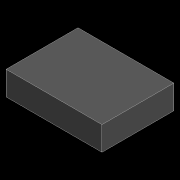
# Autodesk Inventor part: RecieverMockup
Saved by Autodesk Inventor 2022 (Build 260153000, 153)
## iProperties
Created: 2022-09-26
Part Number: RecieverMockup
Material: Generic
Document SubType Name: Modeling
Designer: tandu
Density: 1 g/cm^3
Appearance: Generic
RecieverLongSide: 0.50000000 in
RecieverShortSide: 0.37500000 in
RecieverThickness: 0.12500000 in
Author: tandu
Autodesk Inventor part; units mm, degrees
ref_plane "YZ Plane" through (0, 0, 0) normal (1, 0, 0) x (0, 1, 0)
ref_plane "XZ Plane" through (0, 0, 0) normal (0, 1, 0) x (-1, 0, 0)
ref_plane "XY Plane" through (0, 0, 0) normal (0, 0, 1) x (1, 0, 0)
sketch "Sketch1" plane through (0, 0, 0) normal (0, 1, 0) x (-1, 0, 0)
  line L0 (-6.35, 4.7625) -> (6.35, 4.7625)
  line L1 (6.35, 4.7625) -> (6.35, -4.7625)
  line L2 (6.35, -4.7625) -> (-6.35, -4.7625)
  line L3 (-6.35, -4.7625) -> (-6.35, 4.7625)
  line L4 (-6.35, 4.7625) -> (6.35, -4.7625) construction
  line L5 (6.35, 4.7625) -> (-6.35, -4.7625) construction
  point P0 (0, 0)
  dimension "d0" = 12.7
  dimension "d1" = 9.525
  constraints: 12 end point, 2 midpoint, 2 parallel, 1 horizontal, 1 perpendicular
  measures "d0" distance of L1.end L2.end
  measures "d1" distance of L0.end L1.end
extrude "Extrusion1" add sketch "Sketch1" along normal blind 3.175
equation "\"d0\" = RecieverLongSide"
equation "\"d1\" = RecieverShortSide"
equation "\"d2\" = RecieverThickness"
equation "\"RecieverLongSide\" = 12.7"
equation "\"RecieverShortSide\" = 9.525"
equation "\"RecieverThickness\" = 3.175"
body "Solid1"
